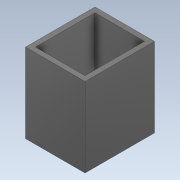
# Autodesk Inventor part: EierkocherTeil2
Saved by Autodesk Inventor 2020 (Build 240168000, 168)
## iProperties
Created: 2022-01-25
Part Number: EierkocherTeil2
Material: Acetalharz, Schwarz
Document SubType Name: Modeling
Designer: Julian Uhl
Density: 1.425 g/cm^3
Appearance: Glatt - Schwarz
Author: Julian Uhl
Autodesk Inventor part; units mm, degrees
ref_plane "YZ Plane" through (0, 0, 0) normal (1, 0, 0) x (0, 1, 0)
ref_plane "XZ Plane" through (0, 0, 0) normal (0, 1, 0) x (-1, 0, 0)
ref_plane "XY Plane" through (0, 0, 0) normal (0, 0, 1) x (1, 0, 0)
sketch "Skizze1" plane through (0, 0, 0) normal (0, 0, 1) x (1, 0, 0)
  line L0 (-24, 0) -> (144, 0) projected
  line L1 (0, -32) -> (0, 192) projected
  line L2 (0, 0) -> (120, 0)
  line L3 (120, 0) -> (120, 160)
  line L4 (120, 160) -> (0, 160)
  line L5 (0, 160) -> (0, 0)
  point P0 (0, 160)
  dimension "d0" = 120
  dimension "d1" = 160
  constraints: 8 end point, 2 parallel, 1 horizontal, 1 perpendicular
  measures "d0" distance between parallel lines of L3 L1
  measures "d1" distance between parallel lines of L2 L4
extrude "Extrusion1" add sketch "Skizze1" along normal blind 140
sketch "Skizze2" plane through (0, 0, 0) normal (0, 0, -1) x (-1, 0, 0)
  line L0 (-10, 10) -> (-110, 10)
  line L1 (-110, 10) -> (-110, 40)
  line L2 (-110, 40) -> (-10, 40)
  line L3 (-10, 40) -> (-10, 10)
  line L4 (0, 0) -> (-120, 0) projected
  line L5 (0, 160) -> (0, 0) projected
  line L6 (-120, 0) -> (-120, 160) projected
  dimension "d4" = 10
  dimension "d5" = 10
  dimension "d6" = 10
  dimension "d7" = 30
  constraints: 8 end point, 2 parallel, 1 horizontal, 1 perpendicular
  measures "d4" distance between parallel lines of L4 L0
  measures "d5" distance between parallel lines of L5 L3
  measures "d6" distance between parallel lines of L6 L1
  measures "d7" distance between parallel lines of L0 L2
extrude "Extrusion2" cut sketch "Skizze2" against normal blind 130
sketch "Skizze3" plane through (0, 160, 0) normal (0, 1, 0) x (1, 0, 0)
  line L0 (110, -130) -> (10, -130)
  line L1 (10, -130) -> (10, -10)
  line L2 (10, -10) -> (110, -10)
  line L3 (110, -10) -> (110, -130)
  line L4 (120, -140) -> (0, -140) projected
  line L5 (0, 0) -> (0, -140) projected
  line L6 (120, 0) -> (120, -140) projected
  line L7 (120, 0) -> (0, 0) projected
  dimension "d10" = 10
  dimension "d11" = 10
  dimension "d12" = 10
  dimension "d13" = 10
  constraints: 8 end point, 2 parallel, 1 horizontal, 1 perpendicular
  measures "d10" distance between parallel lines of L4 L0
  measures "d11" distance between parallel lines of L5 L1
  measures "d12" distance between parallel lines of L6 L3
  measures "d13" distance between parallel lines of L7 L2
extrude "Extrusion3" cut sketch "Skizze3" against normal blind 130 contours L0 L1 L2 L3
